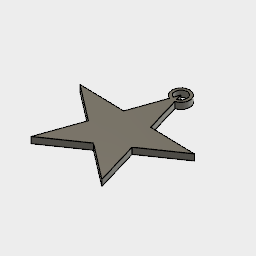
guajian (Autodesk Fusion 360 design; units mm, degrees)
Autodesk Fusion 360 part; units mm, degrees
sketch "草图1" plane through (0, 0, 0) normal (0, 1, 0) x (1, 0, 0)
  line L0 (1.2258, 49.3607) -> (-10.7034, 15.5285)
  line L1 (-18.076, -5.3809) -> (-30.0052, -39.2131)
  line L2 (-46.566, 16.4191) -> (-18.076, -5.3809)
  line L3 (-0.4682, -18.8541) -> (28.0218, -40.6542)
  line L4 (-30.0052, -39.2131) -> (-0.4682, -18.8541)
  line L5 (17.7866, -6.2715) -> (47.3236, 14.0875)
  line L6 (1.2258, 49.3607) -> (11.461, 14.9781)
  line L7 (17.7866, -6.2715) -> (28.0218, -40.6542)
  line L8 (-46.566, 16.4191) -> (-10.7034, 15.5285)
  line L9 (11.461, 14.9781) -> (47.3236, 14.0875)
extrude "拉伸1" add sketch "草图1" along normal blind 5 makes body 1
torus "圆环体基本要素1" add centre line diameter 6.363 section diameter 2.5 placed x (1, 0, 0) y (0, 0, -1) z (0, 1, 0) at (0, 0, -55) separate body makes body 2
delete_face "删除面1" 1 faces at (2.9159, 0.2477, -58.3041) on bodies 2
sketch "草图3" plane through (0, 5, 0) normal (0, 1, 0) x (-1, 0, 0)
  line L0 (-1.2258, -49.3607) -> (10.7034, -15.5285)
  line L1 (10.7034, -15.5285) -> (46.566, -16.4191)
  line L2 (46.566, -16.4191) -> (18.076, 5.3809)
  line L3 (18.076, 5.3809) -> (30.0052, 39.2131)
  line L4 (30.0052, 39.2131) -> (0.4682, 18.8541)
  line L5 (0.4682, 18.8541) -> (-28.0218, 40.6542)
  line L6 (-28.0218, 40.6542) -> (-17.7866, 6.2715)
  line L7 (-17.7866, 6.2715) -> (-47.3236, -14.0875)
  line L8 (-47.3236, -14.0875) -> (-11.461, -14.9781)
  line L9 (-11.461, -14.9781) -> (-1.2258, -49.3607)
  circle A0 centre (-1.2258, -49.3607) radius 4.8494
  circle A1 centre (-1.2258, -49.3607) radius 7.1215
  dimension "d5" = 2.2721
extrude "拉伸2" add sketch "草图3" against normal blind 5 contours L0 L9 A0 A1 picked at (5.1126, -49.7094) bodies 1
